Autodesk Inventor part; units mm, degrees
(part 3 of 4)
  line L942 (14.236161, -150.59225) -> (7.054859, -153.555032)
  spline S133 degree 3 poles (7.054859, -153.555032) (6.871236, -153.625657) (6.716206, -153.668031) (6.603207, -153.668031) (6.166024, -153.668031) (5.855277, -153.315254) (5.855277, -152.849821) (5.855277, -152.511168) (6.06715, -152.229015) (6.448178, -152.073641) knots 9 9 9 9 10 10 10 11 11 11 12 12 12 12
  line L943 (7.054859, -153.555032) -> (6.871236, -153.625657) construction
  line L944 (6.871236, -153.625657) -> (6.716206, -153.668031) construction
  line L945 (6.716206, -153.668031) -> (6.603207, -153.668031) construction
  line L946 (6.603207, -153.668031) -> (6.166024, -153.668031) construction
  line L947 (6.166024, -153.668031) -> (5.855277, -153.315254) construction
  line L948 (5.855277, -153.315254) -> (5.855277, -152.849821) construction
  line L949 (5.855277, -152.849821) -> (5.855277, -152.511168) construction
  line L950 (5.855277, -152.511168) -> (6.06715, -152.229015) construction
  line L951 (6.06715, -152.229015) -> (6.448178, -152.073641) construction
  line L952 (6.448178, -152.073641) -> (8.225847, -151.354305)
  line L953 (8.225847, -151.354305) -> (8.225847, -146.938037)
  line L954 (9.636614, -150.804124) -> (13.770384, -149.181484)
  line L955 (13.770384, -149.181484) -> (13.770384, -149.139109)
  line L956 (13.770384, -149.139109) -> (9.636614, -147.474439)
  line L957 (9.636614, -147.474439) -> (9.636614, -150.804124)
  spline S134 degree 3 poles (14.518314, -153.401381) (14.969621, -153.401381) (15.23765, -153.697659) (15.23765, -154.163436) knots 0 0 0 0 1 1 1 1
  line L958 (14.518314, -153.401381) -> (14.969621, -153.401381) construction
  line L959 (14.969621, -153.401381) -> (15.23765, -153.697659) construction
  line L960 (15.23765, -153.697659) -> (15.23765, -154.163436) construction
  line L961 (15.23765, -154.163436) -> (15.23765, -161.372988)
  spline S135 degree 3 poles (15.23765, -161.372988) (15.23765, -161.83842) (14.969621, -162.120573) (14.518314, -162.120573) (14.080787, -162.120573) (13.812758, -161.83842) (13.812758, -161.372988) knots 2 2 2 2 3 3 3 4 4 4 4
  line L962 (15.23765, -161.372988) -> (15.23765, -161.83842) construction
  line L963 (15.23765, -161.83842) -> (14.969621, -162.120573) construction
  line L964 (14.969621, -162.120573) -> (14.518314, -162.120573) construction
  line L965 (14.518314, -162.120573) -> (14.080787, -162.120573) construction
  line L966 (14.080787, -162.120573) -> (13.812758, -161.83842) construction
  line L967 (13.812758, -161.83842) -> (13.812758, -161.372988) construction
  line L968 (13.812758, -161.372988) -> (13.812758, -158.55111)
  line L969 (13.812758, -158.55111) -> (6.546708, -158.55111)
  spline S136 degree 3 poles (6.546708, -158.55111) (6.137775, -158.55111) (5.855277, -158.226582) (5.855277, -157.775274) (5.855277, -157.323622) (6.137775, -156.999094) (6.546708, -156.999094) knots 6 6 6 6 7 7 7 8 8 8 8
  line L970 (6.546708, -158.55111) -> (6.137775, -158.55111) construction
  line L971 (6.137775, -158.55111) -> (5.855277, -158.226582) construction
  line L972 (5.855277, -158.226582) -> (5.855277, -157.775274) construction
  line L973 (5.855277, -157.775274) -> (5.855277, -157.323622) construction
  line L974 (5.855277, -157.323622) -> (6.137775, -156.999094) construction
  line L975 (6.137775, -156.999094) -> (6.546708, -156.999094) construction
  line L976 (6.546708, -156.999094) -> (13.812758, -156.999094)
  line L977 (13.812758, -156.999094) -> (13.812758, -154.149311)
  spline S137 degree 3 poles (13.812758, -154.149311) (13.812758, -153.697659) (14.080787, -153.401381) (14.518314, -153.401381) knots 10 10 10 10 11 11 11 11
  line L978 (13.812758, -154.149311) -> (13.812758, -153.697659) construction
  line L979 (13.812758, -153.697659) -> (14.080787, -153.401381) construction
  line L980 (14.080787, -153.401381) -> (14.518314, -153.401381) construction
  spline S138 degree 3 poles (10.610198, -162.573603) (13.389701, -162.573603) (15.393024, -164.718175) (15.393024, -167.511803) (15.393024, -170.305431) (13.389701, -172.464128) (10.610198, -172.464128) (7.81657, -172.464128) (5.799122, -170.305431) (5.799122, -167.511803) (5.799122, -164.718175) (7.81657, -162.573603) (10.610198, -162.573603) knots 0 0 0 0 1 1 1 2 2 2 3 3 3 4 4 4 4
  line L981 (10.610198, -162.573603) -> (13.389701, -162.573603) construction
  line L982 (13.389701, -162.573603) -> (15.393024, -164.718175) construction
  line L983 (15.393024, -164.718175) -> (15.393024, -167.511803) construction
  line L984 (15.393024, -167.511803) -> (15.393024, -170.305431) construction
  line L985 (15.393024, -170.305431) -> (13.389701, -172.464128) construction
  line L986 (13.389701, -172.464128) -> (10.610198, -172.464128) construction
  line L987 (10.610198, -172.464128) -> (7.81657, -172.464128) construction
  line L988 (7.81657, -172.464128) -> (5.799122, -170.305431) construction
  line L989 (5.799122, -170.305431) -> (5.799122, -167.511803) construction
  line L990 (5.799122, -167.511803) -> (5.799122, -164.718175) construction
  line L991 (5.799122, -164.718175) -> (7.81657, -162.573603) construction
  line L992 (7.81657, -162.573603) -> (10.610198, -162.573603) construction
  spline S139 degree 3 poles (7.322888, -167.511803) (7.322888, -169.247098) (8.5645, -170.770863) (10.596073, -170.770863) (12.627646, -170.770863) (13.869258, -169.247098) (13.869258, -167.511803) (13.869258, -165.790633) (12.627646, -164.266868) (10.596073, -164.266868) (8.5645, -164.266868) (7.322888, -165.790633) (7.322888, -167.511803) knots 0 0 0 0 1 1 1 2 2 2 3 3 3 4 4 4 4
  line L993 (7.322888, -167.511803) -> (7.322888, -169.247098) construction
  line L994 (7.322888, -169.247098) -> (8.5645, -170.770863) construction
  line L995 (8.5645, -170.770863) -> (10.596073, -170.770863) construction
  line L996 (10.596073, -170.770863) -> (12.627646, -170.770863) construction
  line L997 (12.627646, -170.770863) -> (13.869258, -169.247098) construction
  line L998 (13.869258, -169.247098) -> (13.869258, -167.511803) construction
  line L999 (13.869258, -167.511803) -> (13.869258, -165.790633) construction
  line L1000 (13.869258, -165.790633) -> (12.627646, -164.266868) construction
  line L1001 (12.627646, -164.266868) -> (10.596073, -164.266868) construction
  line L1002 (10.596073, -164.266868) -> (8.5645, -164.266868) construction
  line L1003 (8.5645, -164.266868) -> (7.322888, -165.790633) construction
  line L1004 (7.322888, -165.790633) -> (7.322888, -167.511803) construction
  line L1005 (9.396835, -179.520028) -> (7.153389, -181.763474)
  spline S140 degree 3 poles (7.153389, -181.763474) (6.984235, -181.946753) (6.814736, -182.031503) (6.603207, -182.031503) (6.236304, -182.031503) (5.855277, -181.69285) (5.855277, -181.241198) (5.855277, -180.987294) (5.968276, -180.81814) (6.1519, -180.648641) knots 1 1 1 1 2 2 2 3 3 3 4 4 4 4
  line L1006 (7.153389, -181.763474) -> (6.984235, -181.946753) construction
  line L1007 (6.984235, -181.946753) -> (6.814736, -182.031503) construction
  line L1008 (6.814736, -182.031503) -> (6.603207, -182.031503) construction
  line L1009 (6.603207, -182.031503) -> (6.236304, -182.031503) construction
  line L1010 (6.236304, -182.031503) -> (5.855277, -181.69285) construction
  line L1011 (5.855277, -181.69285) -> (5.855277, -181.241198) construction
  line L1012 (5.855277, -181.241198) -> (5.855277, -180.987294) construction
  line L1013 (5.855277, -180.987294) -> (5.968276, -180.81814) construction
  line L1014 (5.968276, -180.81814) -> (6.1519, -180.648641) construction
  line L1015 (6.1519, -180.648641) -> (9.185306, -177.742359)
  line L1016 (9.185306, -177.742359) -> (9.185306, -176.162093)
  line L1017 (9.185306, -176.162093) -> (6.546708, -176.162093)
  spline S141 degree 3 poles (6.546708, -176.162093) (6.12365, -176.162093) (5.855277, -175.837565) (5.855277, -175.386258) (5.855277, -174.934606) (6.12365, -174.610078) (6.546708, -174.610078) knots 7 7 7 7 8 8 8 9 9 9 9
  line L1018 (6.546708, -176.162093) -> (6.12365, -176.162093) construction
  line L1019 (6.12365, -176.162093) -> (5.855277, -175.837565) construction
  line L1020 (5.855277, -175.837565) -> (5.855277, -175.386258) construction
  line L1021 (5.855277, -175.386258) -> (5.855277, -174.934606) construction
  line L1022 (5.855277, -174.934606) -> (6.12365, -174.610078) construction
  line L1023 (6.12365, -174.610078) -> (6.546708, -174.610078) construction
  line L1024 (6.546708, -174.610078) -> (14.574814, -174.610078)
  spline S142 degree 3 poles (14.574814, -174.610078) (14.983746, -174.610078) (15.23765, -174.864326) (15.23765, -175.315633) knots 10 10 10 10 11 11 11 11
  line L1025 (14.574814, -174.610078) -> (14.983746, -174.610078) construction
  line L1026 (14.983746, -174.610078) -> (15.23765, -174.864326) construction
  line L1027 (15.23765, -174.864326) -> (15.23765, -175.315633) construction
  line L1028 (15.23765, -175.315633) -> (15.23765, -178.221916)
  spline S143 degree 3 poles (15.23765, -178.221916) (15.23765, -180.81814) (13.826883, -181.904379) (12.303118, -181.904379) (11.160379, -181.904379) (9.777863, -181.199168) (9.396835, -179.520028) knots 12 12 12 12 13 13 13 14 14 14 14
  line L1029 (15.23765, -178.221916) -> (15.23765, -180.81814) construction
  line L1030 (15.23765, -180.81814) -> (13.826883, -181.904379) construction
  line L1031 (13.826883, -181.904379) -> (12.303118, -181.904379) construction
  line L1032 (12.303118, -181.904379) -> (11.160379, -181.904379) construction
  line L1033 (11.160379, -181.904379) -> (9.777863, -181.199168) construction
  line L1034 (9.777863, -181.199168) -> (9.396835, -179.520028) construction
  spline S144 degree 3 poles (10.581948, -178.109261) (10.581948, -179.661277) (11.315409, -180.211459) (12.204243, -180.211459) (13.079298, -180.211459) (13.812758, -179.661277) (13.812758, -178.109261) knots 0 0 0 0 1 1 1 2 2 2 2
  line L1035 (10.581948, -178.109261) -> (10.581948, -179.661277) construction
  line L1036 (10.581948, -179.661277) -> (11.315409, -180.211459) construction
  line L1037 (11.315409, -180.211459) -> (12.204243, -180.211459) construction
  line L1038 (12.204243, -180.211459) -> (13.079298, -180.211459) construction
  line L1039 (13.079298, -180.211459) -> (13.812758, -179.661277) construction
  line L1040 (13.812758, -179.661277) -> (13.812758, -178.109261) construction
  line L1041 (13.812758, -178.109261) -> (13.812758, -176.444247)
  spline S145 degree 3 poles (13.812758, -176.444247) (13.812758, -176.246843) (13.728009, -176.162093) (13.48823, -176.162093) knots 3 3 3 3 4 4 4 4
  line L1042 (13.812758, -176.444247) -> (13.812758, -176.246843) construction
  line L1043 (13.812758, -176.246843) -> (13.728009, -176.162093) construction
  line L1044 (13.728009, -176.162093) -> (13.48823, -176.162093) construction
  line L1045 (13.48823, -176.162093) -> (10.581948, -176.162093)
  line L1046 (10.581948, -176.162093) -> (10.581948, -178.109261)
  spline S146 degree 3 poles (5.855277, -187.535387) (5.855277, -187.09786) (6.12365, -186.759552) (6.546708, -186.759552) knots 0 0 0 0 1 1 1 1
  line L1047 (5.855277, -187.535387) -> (5.855277, -187.09786) construction
  line L1048 (5.855277, -187.09786) -> (6.12365, -186.759552) construction
  line L1049 (6.12365, -186.759552) -> (6.546708, -186.759552) construction
  line L1050 (6.546708, -186.759552) -> (9.664863, -186.759552)
  line L1051 (9.664863, -186.759552) -> (14.066662, -183.288618)
  spline S147 degree 3 poles (14.066662, -183.288618) (14.603063, -182.865216) (15.336524, -183.260368) (15.336524, -183.951799) (15.336524, -184.262202) (15.16737, -184.473731) (14.871092, -184.699385) knots 3 3 3 3 4 4 4 5 5 5 5
  line L1052 (14.066662, -183.288618) -> (14.603063, -182.865216) construction
  line L1053 (14.603063, -182.865216) -> (15.336524, -183.260368) construction
  line L1054 (15.336524, -183.260368) -> (15.336524, -183.951799) construction
  line L1055 (15.336524, -183.951799) -> (15.336524, -184.262202) construction
  line L1056 (15.336524, -184.262202) -> (15.16737, -184.473731) construction
  line L1057 (15.16737, -184.473731) -> (14.871092, -184.699385) construction
  line L1058 (14.871092, -184.699385) -> (11.231004, -187.549512)
  line L1059 (11.231004, -187.549512) -> (14.856967, -190.38517)
  spline S148 degree 3 poles (14.856967, -190.38517) (15.153245, -190.625293) (15.336524, -190.794447) (15.336524, -191.147225) (15.336524, -191.838656) (14.574814, -192.219339) (14.038412, -191.782156) knots 7 7 7 7 8 8 8 9 9 9 9
  line L1060 (14.856967, -190.38517) -> (15.153245, -190.625293) construction
  line L1061 (15.153245, -190.625293) -> (15.336524, -190.794447) construction
  line L1062 (15.336524, -190.794447) -> (15.336524, -191.147225) construction
  line L1063 (15.336524, -191.147225) -> (15.336524, -191.838656) construction
  line L1064 (15.336524, -191.838656) -> (14.574814, -192.219339) construction
  line L1065 (14.574814, -192.219339) -> (14.038412, -191.782156) construction
  line L1066 (14.038412, -191.782156) -> (9.678988, -188.311223)
  line L1067 (9.678988, -188.311223) -> (6.546708, -188.311223)
  spline S149 degree 3 poles (6.546708, -188.311223) (6.12365, -188.311223) (5.855277, -187.958789) (5.855277, -187.535387) knots 11 11 11 11 12 12 12 12
  line L1068 (6.546708, -188.311223) -> (6.12365, -188.311223) construction
  line L1069 (6.12365, -188.311223) -> (5.855277, -187.958789) construction
  line L1070 (5.855277, -187.958789) -> (5.855277, -187.535387) construction
  line L1071 (6.400291, -6.445968) -> (12.750291, -6.445968) construction
  line L1072 (46.338938, -27.465197) -> (52.688938, -27.465197) construction
  line L1073 (47.834799, -200.192668) -> (54.184799, -200.192668) construction
  line L1074 (5.855277, -187.958789) -> (12.205277, -187.958789) construction
  line L1075 (1.910163, -1.95584) -> (1.910163, -192.45584)
  line L1076 (1.910163, -192.45584) -> (52.688938, -216.134372)
  line L1077 (52.688938, -216.134372) -> (52.450732, -216.645207)
  line L1078 (1.910163, -1.95584) -> (52.688938, -25.634372)
  line L1079 (1.910163, -1.95584) -> (57.938343, -1.95584) construction
  line L1080 (52.688938, -25.634372) -> (52.688938, -216.134372)
  point P0 (0, 0)
  point P1 (3.752764, -91.883884)
  dimension "d0" = 21.844
  dimension "d8" = 190.5
  dimension "d9" = 115
  dimension "d10" = 25
  constraints: 464 end point, 5 horizontal, 2 coincident, 2 vertical, 1 equal length, 1 perpendicular, 434 other
  measures "d0" distance of L5.start L1075.start
  measures "d8" distance of L1075.start L1075.end
  measures "d9" angle of L1076 L1075
  measures "d10" angle of L1078 L1079
sketch "Sketch1 outline for Extrusion1" plane through (0, 0, 0) normal (0, 1, 0) x (-1, 0, 0)
  line L0 (1.910163, -1.95584) -> (1.910163, -192.45584)
  line L1 (52.688938, -25.634372) -> (1.910163, -1.95584)
  line L2 (1.910163, -192.45584) -> (52.688938, -216.134372)
  line L3 (52.688938, -216.134372) -> (52.688938, -25.634372)
  spline S0 degree 3 poles (14.856967, -190.38517) (15.153245, -190.625293) (15.336524, -190.794447) (15.336524, -191.147225) (15.336524, -191.838656) (14.574814, -192.219339) (14.038412, -191.782156) knots 0 0 0 0 0.5 0.5 0.5 1 1 1 1
  line L4 (11.231004, -187.549512) -> (14.856967, -190.38517)
  line L5 (14.871092, -184.699385) -> (11.231004, -187.549512)
  spline S1 degree 3 poles (14.066662, -183.288618) (14.603063, -182.865216) (15.336524, -183.260368) (15.336524, -183.951799) (15.336524, -184.262202) (15.16737, -184.473731) (14.871092, -184.699385) knots 0 0 0 0 0.5 0.5 0.5 1 1 1 1
  line L6 (9.664863, -186.759552) -> (14.066662, -183.288618)
  line L7 (6.546708, -186.759552) -> (9.664863, -186.759552)
  spline S2 degree 3 poles (5.855277, -187.535387) (5.855277, -187.09786) (6.12365, -186.759552) (6.546708, -186.759552) knots 0 0 0 0 1 1 1 1
  spline S3 degree 3 poles (6.546708, -188.311223) (6.12365, -188.311223) (5.855277, -187.958789) (5.855277, -187.535387) knots 0 0 0 0 1 1 1 1
  line L8 (9.678988, -188.311223) -> (6.546708, -188.311223)
  line L9 (14.038412, -191.782156) -> (9.678988, -188.311223)
  spline S4 degree 3 poles (6.546708, -176.162093) (6.12365, -176.162093) (5.855277, -175.837565) (5.855277, -175.386258) (5.855277, -174.934606) (6.12365, -174.610078) (6.546708, -174.610078) knots 0 0 0 0 0.5 0.5 0.5 1 1 1 1
  line L10 (9.185306, -176.162093) -> (6.546708, -176.162093)
  line L11 (9.185306, -177.742359) -> (9.185306, -176.162093)
  line L12 (6.1519, -180.648641) -> (9.185306, -177.742359)
  spline S5 degree 3 poles (7.153389, -181.763474) (6.984235, -181.946753) (6.814736, -182.031503) (6.603207, -182.031503) (6.236304, -182.031503) (5.855277, -181.69285) (5.855277, -181.241198) (5.855277, -180.987294) (5.968276, -180.81814) (6.1519, -180.648641) knots 0 0 0 0 0.33333333 0.33333333 0.33333333 0.66666667 0.66666667 0.66666667 1 1 1 1
  line L13 (9.396835, -179.520028) -> (7.153389, -181.763474)
  spline S6 degree 3 poles (15.23765, -178.221916) (15.23765, -180.81814) (13.826883, -181.904379) (12.303118, -181.904379) (11.160379, -181.904379) (9.777863, -181.199168) (9.396835, -179.520028) knots 0 0 0 0 0.5 0.5 0.5 1 1 1 1
  line L14 (15.23765, -175.315633) -> (15.23765, -178.221916)
  spline S7 degree 3 poles (14.574814, -174.610078) (14.983746, -174.610078) (15.23765, -174.864326) (15.23765, -175.315633) knots 0 0 0 0 1 1 1 1
  line L15 (6.546708, -174.610078) -> (14.574814, -174.610078)
  spline S8 degree 3 poles (10.610198, -162.573603) (13.389701, -162.573603) (15.393024, -164.718175) (15.393024, -167.511803) (15.393024, -170.305431) (13.389701, -172.464128) (10.610198, -172.464128) (7.81657, -172.464128) (5.799122, -170.305431) (5.799122, -167.511803) (5.799122, -164.718175) (7.81657, -162.573603) (10.610198, -162.573603) knots 0 0 0 0 0.25 0.25 0.25 0.5 0.5 0.5 0.75 0.75 0.75 1 1 1 1
  spline S9 degree 3 poles (13.812758, -154.149311) (13.812758, -153.697659) (14.080787, -153.401381) (14.518314, -153.401381) knots 0 0 0 0 1 1 1 1
  line L16 (13.812758, -156.999094) -> (13.812758, -154.149311)
  line L17 (6.546708, -156.999094) -> (13.812758, -156.999094)
  spline S10 degree 3 poles (6.546708, -158.55111) (6.137775, -158.55111) (5.855277, -158.226582) (5.855277, -157.775274) (5.855277, -157.323622) (6.137775, -156.999094) (6.546708, -156.999094) knots 0 0 0 0 0.5 0.5 0.5 1 1 1 1
  line L18 (13.812758, -158.55111) -> (6.546708, -158.55111)
  line L19 (13.812758, -161.372988) -> (13.812758, -158.55111)
  spline S11 degree 3 poles (15.23765, -161.372988) (15.23765, -161.83842) (14.969621, -162.120573) (14.518314, -162.120573) (14.080787, -162.120573) (13.812758, -161.83842) (13.812758, -161.372988) knots 0 0 0 0 0.5 0.5 0.5 1 1 1 1
  line L20 (15.23765, -154.163436) -> (15.23765, -161.372988)
  spline S12 degree 3 poles (14.518314, -153.401381) (14.969621, -153.401381) (15.23765, -153.697659) (15.23765, -154.163436) knots 0 0 0 0 1 1 1 1
  line L21 (8.225847, -146.938037) -> (6.434053, -146.204577)
  line L22 (8.225847, -151.354305) -> (8.225847, -146.938037)
  line L23 (6.448178, -152.073641) -> (8.225847, -151.354305)
  spline S13 degree 3 poles (7.054859, -153.555032) (6.871236, -153.625657) (6.716206, -153.668031) (6.603207, -153.668031) (6.166024, -153.668031) (5.855277, -153.315254) (5.855277, -152.849821) (5.855277, -152.511168) (6.06715, -152.229015) (6.448178, -152.073641) knots 0 0 0 0 0.33333333 0.33333333 0.33333333 0.66666667 0.66666667 0.66666667 1 1 1 1
  line L24 (14.236161, -150.59225) -> (7.054859, -153.555032)
  spline S14 degree 3 poles (15.322399, -149.209733) (15.322399, -149.858789) (15.026121, -150.267722) (14.236161, -150.59225) knots 0 0 0 0 1 1 1 1
  line L25 (15.322399, -149.110859) -> (15.322399, -149.209733)
  spline S15 degree 3 poles (14.236161, -147.742467) (15.026121, -148.05287) (15.322399, -148.475928) (15.322399, -149.110859) knots 0 0 0 0 1 1 1 1
  line L26 (7.111014, -144.779685) -> (14.236161, -147.742467)
  spline S16 degree 3 poles (6.560832, -144.652561) (6.744456, -144.638436) (6.91361, -144.694936) (7.111014, -144.779685) knots 0 0 0 0 1 1 1 1
  spline S17 degree 3 poles (6.434053, -146.204577) (6.053025, -146.049203) (5.855277, -145.809424) (5.855277, -145.442521) (5.855277, -144.991214) (6.1519, -144.680811) (6.560832, -144.652561) knots 0 0 0 0 0.5 0.5 0.5 1 1 1 1
  line L27 (9.396835, -140.799222) -> (7.153389, -143.042668)
  spline S18 degree 3 poles (15.23765, -139.501454) (15.23765, -142.097334) (13.826883, -143.183572) (12.303118, -143.183572) (11.160379, -143.183572) (9.777863, -142.478361) (9.396835, -140.799222) knots 0 0 0 0 0.5 0.5 0.5 1 1 1 1
  line L28 (15.23765, -136.594827) -> (15.23765, -139.501454)
  spline S19 degree 3 poles (14.574814, -135.889616) (14.983746, -135.889616) (15.23765, -136.14352) (15.23765, -136.594827) knots 0 0 0 0 1 1 1 1
  line L29 (6.546708, -135.889616) -> (14.574814, -135.889616)
  spline S20 degree 3 poles (6.546708, -137.441632) (6.12365, -137.441632) (5.855277, -137.117104) (5.855277, -136.665452) (5.855277, -136.214144) (6.12365, -135.889616) (6.546708, -135.889616) knots 0 0 0 0 0.5 0.5 0.5 1 1 1 1
  line L30 (9.185306, -137.441632) -> (6.546708, -137.441632)
  line L31 (9.185306, -139.021553) -> (9.185306, -137.441632)
  line L32 (6.1519, -141.92818) -> (9.185306, -139.021553)
  spline S21 degree 3 poles (7.153389, -143.042668) (6.984235, -143.225947) (6.814736, -143.310696) (6.603207, -143.310696) (6.236304, -143.310696) (5.855277, -142.972044) (5.855277, -142.520736) (5.855277, -142.266832) (5.968276, -142.097334) (6.1519, -141.92818) knots 0 0 0 0 0.33333333 0.33333333 0.33333333 0.66666667 0.66666667 0.66666667 1 1 1 1
  spline S22 degree 3 poles (10.610198, -123.853142) (13.389701, -123.853142) (15.393024, -125.997714) (15.393024, -128.790997) (15.393024, -131.584625) (13.389701, -133.743322) (10.610198, -133.743322) (7.81657, -133.743322) (5.799122, -131.584625) (5.799122, -128.790997) (5.799122, -125.997714) (7.81657, -123.853142) (10.610198, -123.853142) knots 0 0 0 0 0.25 0.25 0.25 0.5 0.5 0.5 0.75 0.75 0.75 1 1 1 1
  spline S23 degree 3 poles (5.954151, -115.696706) (5.954151, -115.245226) (6.208055, -114.991322) (6.631457, -114.991322) knots 0 0 0 0 1 1 1 1
  line L33 (5.954151, -119.068593) -> (5.954151, -115.696706)
  spline S24 degree 3 poles (10.553698, -120.747733) (10.215045, -121.819846) (9.35446, -122.355903) (8.493876, -122.355903) (7.040734, -122.355903) (5.954151, -121.19904) (5.954151, -119.068593) knots 0 0 0 0 0.5 0.5 0.5 1 1 1 1
  spline S25 degree 3 poles (15.23765, -118.70169) (15.23765, -120.959261) (14.123162, -122.102) (12.599396, -122.102) (11.668186, -122.102) (10.864101, -121.509443) (10.553698, -120.747733) knots 0 0 0 0 0.5 0.5 0.5 1 1 1 1
  line L34 (15.23765, -115.696706) -> (15.23765, -118.70169)
  spline S26 degree 3 poles (14.574814, -114.991322) (14.983746, -114.991322) (15.23765, -115.245226) (15.23765, -115.696706) knots 0 0 0 0 1 1 1 1
  line L35 (6.631457, -114.991322) -> (14.574814, -114.991322)
  line L36 (29.80093, -191.867595) -> (23.480041, -191.867595)
  line L37 (23.494166, -196.368267) -> (29.80093, -191.867595)
  spline S27 degree 3 poles (22.788955, -197.51135) (22.788955, -197.031448) (23.000484, -196.721045) (23.494166, -196.368267) knots 0 0 0 0 1 1 1 1
  line L38 (22.788955, -197.567505) -> (22.788955, -197.51135)
  spline S28 degree 3 poles (23.62129, -198.498714) (23.127263, -198.498714) (22.788955, -198.061532) (22.788955, -197.567505) knots 0 0 0 0 1 1 1 1
  line L39 (31.578599, -198.498714) -> (23.62129, -198.498714)
  spline S29 degree 3 poles (31.578599, -196.946699) (31.987876, -196.946699) (32.27003, -197.271227) (32.27003, -197.722879) (32.27003, -198.174187) (31.987876, -198.498714) (31.578599, -198.498714) knots 0 0 0 0 0.5 0.5 0.5 1 1 1 1
  line L40 (25.356757, -196.946699) -> (31.578599, -196.946699)
  line L41 (31.479897, -192.446026) -> (25.356757, -196.946699)
  spline S30 degree 3 poles (32.255905, -191.260913) (32.255905, -191.740815) (32.086578, -191.994719) (31.479897, -192.446026) knots 0 0 0 0 1 1 1 1
  line L42 (32.255905, -191.176509) -> (32.255905, -191.260913)
  spline S31 degree 3 poles (31.324696, -190.315579) (31.889002, -190.315579) (32.255905, -190.696607) (32.255905, -191.176509) knots 0 0 0 0 1 1 1 1
  line L43 (23.480041, -190.315579) -> (31.324696, -190.315579)
  spline S32 degree 3 poles (23.480041, -191.867595) (23.071108, -191.867595) (22.788955, -191.543067) (22.788955, -191.091759) (22.788955, -190.640107) (23.071108, -190.315579) (23.480041, -190.315579) knots 0 0 0 0 0.5 0.5 0.5 1 1 1 1
  spline S33 degree 3 poles (27.543531, -178.279105) (30.323034, -178.279105) (32.326357, -180.423677) (32.326357, -183.217304) (32.326357, -186.010932) (30.323034, -188.169629) (27.543531, -188.169629) (24.750075, -188.169629) (22.732455, -186.010932) (22.732455, -183.217304) (22.732455, -180.423677) (24.750075, -178.279105) (27.543531, -178.279105) knots 0 0 0 0 0.25 0.25 0.25 0.5 0.5 0.5 0.75 0.75 0.75 1 1 1 1
  spline S34 degree 3 poles (31.578599, -174.595953) (31.987876, -174.595953) (32.27003, -174.920481) (32.27003, -175.372133) knots 0 0 0 0 1 1 1 1
  line L44 (23.480041, -174.595953) -> (31.578599, -174.595953)
  spline S35 degree 3 poles (23.480041, -176.147969) (23.071108, -176.147969) (22.788955, -175.823441) (22.788955, -175.372133) (22.788955, -174.920481) (23.071108, -174.595953) (23.480041, -174.595953) knots 0 0 0 0 0.5 0.5 0.5 1 1 1 1
  line L45 (31.578599, -176.147969) -> (23.480041, -176.147969)
  spline S36 degree 3 poles (32.27003, -175.372133) (32.27003, -175.823441) (31.987876, -176.147969) (31.578599, -176.147969) knots 0 0 0 0 1 1 1 1
  line L46 (30.746264, -169.444846) -> (23.480041, -169.444846)
  line L47 (30.746264, -172.266724) -> (30.746264, -169.444846)
  spline S37 degree 3 poles (32.171155, -172.266724) (32.171155, -172.732156) (31.903127, -173.01431) (31.451647, -173.01431) (31.014292, -173.01431) (30.746264, -172.732156) (30.746264, -172.266724) knots 0 0 0 0 0.5 0.5 0.5 1 1 1 1
  line L48 (32.171155, -165.057173) -> (32.171155, -172.266724)
  spline S38 degree 3 poles (31.451647, -164.295117) (31.903127, -164.295117) (32.171155, -164.591396) (32.171155, -165.057173) knots 0 0 0 0 1 1 1 1
  spline S39 degree 3 poles (30.746264, -165.043048) (30.746264, -164.591396) (31.014292, -164.295117) (31.451647, -164.295117) knots 0 0 0 0 1 1 1 1
  line L49 (30.746264, -167.892831) -> (30.746264, -165.043048)
  line L50 (23.480041, -167.892831) -> (30.746264, -167.892831)
  spline S40 degree 3 poles (23.480041, -169.444846) (23.071108, -169.444846) (22.788955, -169.120318) (22.788955, -168.669011) (22.788955, -168.217359) (23.071108, -167.892831) (23.480041, -167.892831) knots 0 0 0 0 0.5 0.5 0.5 1 1 1 1
  line L51 (25.15918, -162.248042) -> (25.15918, -157.831774)
  line L52 (23.381511, -162.967378) -> (25.15918, -162.248042)
  spline S41 degree 3 poles (23.988192, -164.448769) (23.804569, -164.519393) (23.64954, -164.561768) (23.53654, -164.561768) (23.099358, -164.561768) (22.788955, -164.20899) (22.788955, -163.743558) (22.788955, -163.404905) (23.000484, -163.122752) (23.381511, -162.967378) knots 0 0 0 0 0.33333333 0.33333333 0.33333333 0.66666667 0.66666667 0.66666667 1 1 1 1
  line L53 (31.169494, -161.485987) -> (23.988192, -164.448769)
  spline S42 degree 3 poles (32.255905, -160.10347) (32.255905, -160.752526) (31.959627, -161.161459) (31.169494, -161.485987) knots 0 0 0 0 1 1 1 1
  line L54 (32.255905, -160.004596) -> (32.255905, -160.10347)
  spline S43 degree 3 poles (31.169494, -158.636204) (31.959627, -158.946607) (32.255905, -159.369664) (32.255905, -160.004596) knots 0 0 0 0 1 1 1 1
  line L55 (24.044348, -155.673422) -> (31.169494, -158.636204)
  spline S44 degree 3 poles (23.494166, -155.546298) (23.677789, -155.532173) (23.846944, -155.588672) (24.044348, -155.673422) knots 0 0 0 0 1 1 1 1
  spline S45 degree 3 poles (23.367386, -157.098313) (22.986359, -156.942939) (22.788955, -156.703161) (22.788955, -156.336258) (22.788955, -155.88495) (23.085233, -155.574547) (23.494166, -155.546298) knots 0 0 0 0 0.5 0.5 0.5 1 1 1 1
  line L56 (25.15918, -157.831774) -> (23.367386, -157.098313)
  spline S46 degree 3 poles (48.511932, -199.684861) (48.356731, -199.938764) (48.159327, -200.192668) (47.834799, -200.192668) (47.453771, -200.192668) (47.072916, -199.952889) (47.072916, -199.515707) (47.072916, -199.289708) (47.129243, -199.148804) (47.242242, -198.937275) (47.524396, -198.344374) (47.792424, -197.540289) (47.792424, -196.679704) (47.792424, -195.325437) (47.171618, -194.577507) (46.466235, -194.577507) (45.520901, -194.577507) (45.281122, -195.494591) (44.956594, -197.159261) (44.617941, -198.866651) (44.251211, -200.418666) (42.360542, -200.418666) (40.879151, -200.418666) (39.651664, -199.02168) (39.651664, -196.707954) (39.651664, -195.212438) (40.117268, -193.815796) (40.596998, -193.081991) (40.794574, -192.799838) (41.048478, -192.729213) (41.231929, -192.729213) (41.641034, -192.729213) (42.036014, -193.039616) (42.036014, -193.448894) (42.036014, -193.646298) (41.951437, -193.843701) (41.852563, -194.04145) (41.457583, -194.83141) (41.161304, -195.790869) (41.161304, -196.792703) (41.161304, -198.076346) (41.626909, -198.767776) (42.332292, -198.767776) (43.1083, -198.767776) (43.305876, -198.020191) (43.644529, -196.312801) (43.98301, -194.591632) (44.364037, -192.926617) (46.437985, -192.926617) (47.877001, -192.926617) (49.25969, -194.238854) (49.25969, -196.750329) (49.25969, -198.006066) (48.808211, -199.191179) (48.511932, -199.684861) knots 0 0 0 0 0.05555556 0.05555556 0.05555556 0.11111111 0.11111111 0.11111111 0.16666667 0.16666667 0.16666667 0.22222222 0.22222222 0.22222222 0.27777778 0.27777778 0.27777778 0.33333333 0.33333333 0.33333333 0.38888889 0.38888889 0.38888889 0.44444444 0.44444444 0.44444444 0.5 0.5 0.5 0.55555556 0.55555556 0.55555556 0.61111111 0.61111111 0.61111111 0.66666667 0.66666667 0.66666667 0.72222222 0.72222222 0.72222222 0.77777778 0.77777778 0.77777778 0.83333333 0.83333333 0.83333333 0.88888889 0.88888889 0.88888889 0.94444444 0.94444444 0.94444444 1 1 1 1
  line L57 (48.511932, -184.121298) -> (43.785606, -184.121298)
  spline S47 degree 3 poles (48.511932, -182.569282) (48.92121, -182.569282) (49.203363, -182.89381) (49.203363, -183.345117) (49.203363, -183.79677) (48.92121, -184.121298) (48.511932, -184.121298) knots 0 0 0 0 0.5 0.5 0.5 1 1 1 1
  line L58 (43.700857, -182.569282) -> (48.511932, -182.569282)
  spline S48 degree 3 poles (43.700857, -190.582919) (41.358881, -190.582919) (39.637539, -189.087403) (39.637539, -186.575928) (39.637539, -184.050673) (41.358881, -182.569282) (43.700857, -182.569282) knots 0 0 0 0 0.5 0.5 0.5 1 1 1 1
  line L59 (48.511932, -190.582919) -> (43.700857, -190.582919)
  spline S49 degree 3 poles (48.511932, -189.030903) (48.92121, -189.030903) (49.203363, -189.355431) (49.203363, -189.807083) (49.203363, -190.258391) (48.92121, -190.582919) (48.511932, -190.582919) knots 0 0 0 0 0.5 0.5 0.5 1 1 1 1
  line L60 (43.785606, -189.030903) -> (48.511932, -189.030903)
  spline S50 degree 3 poles (41.14718, -186.575928) (41.14718, -188.085569) (42.177091, -189.030903) (43.785606, -189.030903) knots 0 0 0 0 1 1 1 1
  spline S51 degree 3 poles (43.785606, -184.121298) (42.191216, -184.121298) (41.14718, -185.052162) (41.14718, -186.575928) knots 0 0 0 0 1 1 1 1
  spline S52 degree 3 poles (44.476864, -170.617212) (47.256367, -170.617212) (49.25969, -172.761784) (49.25969, -175.555412) (49.25969, -178.34904) (47.256367, -180.507737) (44.476864, -180.507737) (41.683409, -180.507737) (39.665788, -178.34904) (39.665788, -175.555412) (39.665788, -172.761784) (41.683409, -170.617212) (44.476864, -170.617212) knots 0 0 0 0 0.25 0.25 0.25 0.5 0.5 0.5 0.75 0.75 0.75 1 1 1 1
  line L61 (46.706013, -166.890652) -> (43.729106, -164.858735)
  line L62 (46.706013, -166.918902) -> (46.706013, -166.890652)
  line L63 (40.413546, -166.918902) -> (46.706013, -166.918902)
  spline S53 degree 3 poles (40.413546, -168.470918) (39.990316, -168.470918) (39.722288, -168.14639) (39.722288, -167.694738) (39.722288, -167.24343) (39.990316, -166.918902) (40.413546, -166.918902) knots 0 0 0 0 0.5 0.5 0.5 1 1 1 1
  line L64 (48.286279, -168.470918) -> (40.413546, -168.470918)
  spline S54 degree 3 poles (49.189238, -167.567958) (49.189238, -168.075765) (48.83646, -168.470918) (48.286279, -168.470918) knots 0 0 0 0 1 1 1 1
  line L65 (49.189238, -167.454959) -> (49.189238, -167.567958)
  spline S55 degree 3 poles (48.455605, -166.36872) (48.86471, -166.650874) (49.189238, -166.918902) (49.189238, -167.454959) knots 0 0 0 0 1 1 1 1
  line L66 (44.998969, -164.0264) -> (48.455605, -166.36872)
  line L67 (44.998969, -164.012275) -> (44.998969, -164.0264)
  line L68 (48.44148, -161.656174) -> (44.998969, -164.012275)
  spline S56 degree 3 poles (49.189238, -160.499311) (49.189238, -161.035368) (48.86471, -161.374021) (48.44148, -161.656174) knots 0 0 0 0 1 1 1 1
  line L69 (49.189238, -160.386312) -> (49.189238, -160.499311)
  spline S57 degree 3 poles (48.286279, -159.469228) (48.83646, -159.469228) (49.189238, -159.86438) (49.189238, -160.386312) knots 0 0 0 0 1 1 1 1
  line L70 (40.413546, -159.469228) -> (48.286279, -159.469228)
  spline S58 degree 3 poles (40.413546, -161.021243) (39.990316, -161.021243) (39.722288, -160.696715) (39.722288, -160.245408) (39.722288, -159.793756) (39.990316, -159.469228) (40.413546, -159.469228) knots 0 0 0 0 0.5 0.5 0.5 1 1 1 1
  line L71 (46.706013, -161.021243) -> (40.413546, -161.021243)
  line L72 (46.706013, -161.063618) -> (46.706013, -161.021243)
  line L73 (43.729106, -163.095191) -> (46.706013, -161.063618)
  spline S59 degree 3 poles (43.729106, -164.858735) (43.305876, -164.576582) (43.13655, -164.350928) (43.13655, -163.9699) (43.13655, -163.602998) (43.305876, -163.391469) (43.729106, -163.095191) knots 0 0 0 0 0.5 0.5 0.5 1 1 1 1
  line L74 (31.578599, -149.53495) -> (24.651201, -149.53495)
  spline S60 degree 3 poles (32.255905, -148.75877) (32.255905, -149.210422) (31.987876, -149.53495) (31.578599, -149.53495) knots 0 0 0 0 1 1 1 1
  spline S61 degree 3 poles (31.578599, -147.982935) (31.987876, -147.982935) (32.255905, -148.307463) (32.255905, -148.75877) knots 0 0 0 0 1 1 1 1
  line L75 (23.607165, -147.982935) -> (31.578599, -147.982935)
  spline S62 degree 3 poles (22.887484, -148.744645) (22.887484, -148.279213) (23.141388, -147.982935) (23.607165, -147.982935) knots 0 0 0 0 1 1 1 1
  line L76 (22.887484, -153.936749) -> (22.887484, -148.744645)
  spline S63 degree 3 poles (24.326501, -153.936749) (24.326501, -154.402181) (24.058472, -154.684335) (23.607165, -154.684335) (23.155513, -154.684335) (22.887484, -154.402181) (22.887484, -153.936749) knots 0 0 0 0 0.5 0.5 0.5 1 1 1 1
  line L77 (24.326501, -149.817104) -> (24.326501, -153.936749)
  spline S64 degree 3 poles (24.651201, -149.53495) (24.397125, -149.53495) (24.326501, -149.619355) (24.326501, -149.817104) knots 0 0 0 0 1 1 1 1
  spline S65 degree 3 poles (24.213846, -141.321843) (24.213846, -142.831484) (25.243757, -143.776818) (26.852273, -143.776818) knots 0 0 0 0 1 1 1 1
  spline S66 degree 3 poles (26.852273, -138.866868) (25.257882, -138.866868) (24.213846, -139.798077) (24.213846, -141.321843) knots 0 0 0 0 1 1 1 1
  line L78 (31.578599, -138.866868) -> (26.852273, -138.866868)
  spline S67 degree 3 poles (31.578599, -137.314852) (31.987876, -137.314852) (32.27003, -137.63938) (32.27003, -138.090688) (32.27003, -138.54234) (31.987876, -138.866868) (31.578599, -138.866868) knots 0 0 0 0 0.5 0.5 0.5 1 1 1 1
  line L79 (26.767523, -137.314852) -> (31.578599, -137.314852)
  spline S68 degree 3 poles (26.767523, -145.328489) (24.425375, -145.328489) (22.704205, -143.832973) (22.704205, -141.321843) (22.704205, -138.796243) (24.425375, -137.314852) (26.767523, -137.314852) knots 0 0 0 0 0.5 0.5 0.5 1 1 1 1
  line L80 (31.578599, -145.328489) -> (26.767523, -145.328489)
  spline S69 degree 3 poles (31.578599, -143.776818) (31.987876, -143.776818) (32.27003, -144.101001) (32.27003, -144.552653) (32.27003, -145.003961) (31.987876, -145.328489) (31.578599, -145.328489) knots 0 0 0 0 0.5 0.5 0.5 1 1 1 1
  line L81 (26.852273, -143.776818) -> (31.578599, -143.776818)
  line L82 (29.77268, -133.108735) -> (29.77268, -133.080485)
  line L83 (23.480041, -133.108735) -> (29.77268, -133.108735)
  spline S70 degree 3 poles (23.480041, -134.660751) (23.056983, -134.660751) (22.788955, -134.336223) (22.788955, -133.884571) (22.788955, -133.433263) (23.056983, -133.108735) (23.480041, -133.108735) knots 0 0 0 0 0.5 0.5 0.5 1 1 1 1
  line L84 (31.352945, -134.660751) -> (23.480041, -134.660751)
  spline S71 degree 3 poles (32.255905, -133.757791) (32.255905, -134.265598) (31.903127, -134.660751) (31.352945, -134.660751) knots 0 0 0 0 1 1 1 1
  line L85 (32.255905, -133.644792) -> (32.255905, -133.757791)
  spline S72 degree 3 poles (31.522272, -132.558553) (31.931377, -132.840707) (32.255905, -133.108735) (32.255905, -133.644792) knots 0 0 0 0 1 1 1 1
  line L86 (28.065635, -130.216577) -> (31.522272, -132.558553)
  line L87 (28.065635, -130.202453) -> (28.065635, -130.216577)
  line L88 (31.508147, -127.846007) -> (28.065635, -130.202453)
  spline S73 degree 3 poles (32.255905, -126.689144) (32.255905, -127.225546) (31.931377, -127.563854) (31.508147, -127.846007) knots 0 0 0 0 1 1 1 1
  line L89 (32.255905, -126.57649) -> (32.255905, -126.689144)
  spline S74 degree 3 poles (31.352945, -125.659405) (31.903127, -125.659405) (32.255905, -126.054213) (32.255905, -126.57649) knots 0 0 0 0 1 1 1 1
  line L90 (23.480041, -125.659405) -> (31.352945, -125.659405)
  spline S75 degree 3 poles (23.480041, -127.211421) (23.056983, -127.211421) (22.788955, -126.886893) (22.788955, -126.435241) (22.788955, -125.983933) (23.056983, -125.659405) (23.480041, -125.659405) knots 0 0 0 0 0.5 0.5 0.5 1 1 1 1
  line L91 (29.77268, -127.211421) -> (23.480041, -127.211421)
  line L92 (29.77268, -127.253451) -> (29.77268, -127.211421)
  line L93 (26.795773, -129.285368) -> (29.77268, -127.253451)
  spline S76 degree 3 poles (26.795773, -131.048913) (26.372543, -130.766759) (26.203217, -130.540761) (26.203217, -130.160078) (26.203217, -129.793175) (26.372543, -129.581646) (26.795773, -129.285368) knots 0 0 0 0 0.5 0.5 0.5 1 1 1 1
  line L94 (29.77268, -133.080485) -> (26.795773, -131.048913)
  line L95 (26.118639, -119.196062) -> (26.118639, -117.615968)
  line L96 (23.085233, -122.102344) -> (26.118639, -119.196062)
  spline S77 degree 3 poles (24.086722, -123.216832) (23.917568, -123.400456) (23.748069, -123.485205) (23.53654, -123.485205) (23.169638, -123.485205) (22.788955, -123.146553) (22.788955, -122.6949) (22.788955, -122.440997) (22.901609, -122.271843) (23.085233, -122.102344) knots 0 0 0 0 0.33333333 0.33333333 0.33333333 0.66666667 0.66666667 0.66666667 1 1 1 1
  line L97 (26.330168, -120.973731) -> (24.086722, -123.216832)
  spline S78 degree 3 poles (32.171155, -119.675619) (32.171155, -122.271843) (30.760389, -123.358081) (29.236623, -123.358081) (28.093713, -123.358081) (26.711196, -122.652526) (26.330168, -120.973731) knots 0 0 0 0 0.5 0.5 0.5 1 1 1 1
  line L98 (32.171155, -116.769336) -> (32.171155, -119.675619)
  spline S79 degree 3 poles (31.508147, -116.063953) (31.917252, -116.063953) (32.171155, -116.317856) (32.171155, -116.769336) knots 0 0 0 0 1 1 1 1
  line L99 (23.480041, -116.063953) -> (31.508147, -116.063953)
  spline S80 degree 3 poles (23.480041, -117.615968) (23.056983, -117.615968) (22.788955, -117.29144) (22.788955, -116.839961) (22.788955, -116.388481) (23.056983, -116.063953) (23.480041, -116.063953) knots 0 0 0 0 0.5 0.5 0.5 1 1 1 1
  line L100 (26.118639, -117.615968) -> (23.480041, -117.615968)
  spline S81 degree 3 poles (44.476864, -147.432753) (47.256367, -147.432753) (49.25969, -149.577325) (49.25969, -152.370953) (49.25969, -155.164236) (47.256367, -157.322933) (44.476864, -157.322933) (41.683409, -157.322933) (39.665788, -155.164236) (39.665788, -152.370953) (39.665788, -149.577325) (41.683409, -147.432753) (44.476864, -147.432753) knots 0 0 0 0 0.25 0.25 0.25 0.5 0.5 0.5 0.75 0.75 0.75 1 1 1 1
  spline S82 degree 3 poles (40.413546, -138.655683) (40.004441, -138.655683) (39.722288, -138.331155) (39.722288, -137.879503) (39.722288, -137.428196) (40.004441, -137.103668) (40.413546, -137.103668) knots 0 0 0 0 0.5 0.5 0.5 1 1 1 1
  line L101 (46.734263, -138.655683) -> (40.413546, -138.655683)
  line L102 (40.427671, -143.156356) -> (46.734263, -138.655683)
  spline S83 degree 3 poles (39.722288, -144.299094) (39.722288, -143.819192) (39.933817, -143.508789) (40.427671, -143.156356) knots 0 0 0 0 1 1 1 1
  line L103 (39.722288, -144.355594) -> (39.722288, -144.299094)
  spline S84 degree 3 poles (40.554623, -145.286803) (40.060769, -145.286803) (39.722288, -144.849276) (39.722288, -144.355594) knots 0 0 0 0 1 1 1 1
  line L104 (48.511932, -145.286803) -> (40.554623, -145.286803)
  spline S85 degree 3 poles (48.511932, -143.734788) (48.92121, -143.734788) (49.203363, -144.059316) (49.203363, -144.510623) (49.203363, -144.962275) (48.92121, -145.286803) (48.511932, -145.286803) knots 0 0 0 0 0.5 0.5 0.5 1 1 1 1
  line L105 (42.29009, -143.734788) -> (48.511932, -143.734788)
  line L106 (48.41323, -139.234115) -> (42.29009, -143.734788)
  spline S86 degree 3 poles (49.189238, -138.049002) (49.189238, -138.528559) (49.019912, -138.782463) (48.41323, -139.234115) knots 0 0 0 0 1 1 1 1
  line L107 (49.189238, -137.964253) -> (49.189238, -138.049002)
  spline S87 degree 3 poles (48.258029, -137.103668) (48.822336, -137.103668) (49.189238, -137.484351) (49.189238, -137.964253) knots 0 0 0 0 1 1 1 1
  line L108 (40.413546, -137.103668) -> (48.258029, -137.103668)
  spline S88 degree 3 poles (44.476864, -125.067193) (47.256367, -125.067193) (49.25969, -127.211765) (49.25969, -130.005049) (49.25969, -132.798677) (47.256367, -134.957373) (44.476864, -134.957373) (41.683409, -134.957373) (39.665788, -132.798677) (39.665788, -130.005049) (39.665788, -127.211765) (41.683409, -125.067193) (44.476864, -125.067193) knots 0 0 0 0 0.25 0.25 0.25 0.5 0.5 0.5 0.75 0.75 0.75 1 1 1 1
  spline S89 degree 3 poles (47.679597, -116.642901) (47.679597, -116.191421) (47.947626, -115.895143) (48.384981, -115.895143) knots 0 0 0 0 1 1 1 1
  line L109 (47.679597, -119.492684) -> (47.679597, -116.642901)
  line L110 (40.413546, -119.492684) -> (47.679597, -119.492684)
  spline S90 degree 3 poles (40.413546, -121.0447) (40.004441, -121.0447) (39.722288, -120.720172) (39.722288, -120.268864) (39.722288, -119.817212) (40.004441, -119.492684) (40.413546, -119.492684) knots 0 0 0 0 0.5 0.5 0.5 1 1 1 1
  line L111 (47.679597, -121.0447) -> (40.413546, -121.0447)
  line L112 (47.679597, -123.866577) -> (47.679597, -121.0447)
  spline S91 degree 3 poles (49.104489, -123.866577) (49.104489, -124.33201) (48.83646, -124.614163) (48.384981, -124.614163) (47.947626, -124.614163) (47.679597, -124.33201) (47.679597, -123.866577) knots 0 0 0 0 0.5 0.5 0.5 1 1 1 1
  line L113 (49.104489, -116.657026) -> (49.104489, -123.866577)
  spline S92 degree 3 poles (48.384981, -115.895143) (48.83646, -115.895143) (49.104489, -116.191421) (49.104489, -116.657026) knots 0 0 0 0 1 1 1 1
  spline S93 degree 3 poles (14.236161, -107.17354) (15.026121, -107.483943) (15.322399, -107.907173) (15.322399, -108.542104) knots 0 0 0 0 1 1 1 1
  line L114 (7.111014, -104.210757) -> (14.236161, -107.17354)
  spline S94 degree 3 poles (6.560832, -104.083633) (6.744456, -104.069681) (6.91361, -104.126008) (7.111014, -104.210757) knots 0 0 0 0 1 1 1 1
  spline S95 degree 3 poles (6.434053, -105.635649) (6.053025, -105.480447) (5.855277, -105.240669) (5.855277, -104.873766) (5.855277, -104.422286) (6.1519, -104.111883) (6.560832, -104.083633) knots 0 0 0 0 0.5 0.5 0.5 1 1 1 1
  line L115 (8.225847, -106.369282) -> (6.434053, -105.635649)
  line L116 (8.225847, -110.785378) -> (8.225847, -106.369282)
  line L117 (6.448178, -111.504886) -> (8.225847, -110.785378)
  spline S96 degree 3 poles (7.054859, -112.986277) (6.871236, -113.056901) (6.716206, -113.099276) (6.603207, -113.099276) (6.166024, -113.099276) (5.855277, -112.746498) (5.855277, -112.280894) (5.855277, -111.942241) (6.06715, -111.660087) (6.448178, -111.504886) knots 0 0 0 0 0.33333333 0.33333333 0.33333333 0.66666667 0.66666667 0.66666667 1 1 1 1
  line L118 (14.236161, -110.023495) -> (7.054859, -112.986277)
  spline S97 degree 3 poles (15.322399, -108.640806) (15.322399, -109.289862) (15.026121, -109.698967) (14.236161, -110.023495) knots 0 0 0 0 1 1 1 1
  line L119 (15.322399, -108.542104) -> (15.322399, -108.640806)
  line L120 (6.673832, -96.520271) -> (14.645093, -96.520271)
  spline S98 degree 3 poles (5.954151, -97.282154) (5.954151, -96.816549) (6.208055, -96.520271) (6.673832, -96.520271) knots 0 0 0 0 1 1 1 1
  line L121 (5.954151, -102.474085) -> (5.954151, -97.282154)
  spline S99 degree 3 poles (7.393167, -102.474085) (7.393167, -102.939689) (7.125139, -103.221843) (6.673832, -103.221843) (6.22218, -103.221843) (5.954151, -102.939689) (5.954151, -102.474085) knots 0 0 0 0 0.5 0.5 0.5 1 1 1 1
  line L122 (7.393167, -98.35444) -> (7.393167, -102.474085)
  spline S100 degree 3 poles (7.717695, -98.072286) (7.463792, -98.072286) (7.393167, -98.156863) (7.393167, -98.35444) knots 0 0 0 0 1 1 1 1
  line L123 (14.645093, -98.072286) -> (7.717695, -98.072286)
  spline S101 degree 3 poles (15.322399, -97.296279) (15.322399, -97.747758) (15.054371, -98.072286) (14.645093, -98.072286) knots 0 0 0 0 1 1 1 1
  spline S102 degree 3 poles (14.645093, -96.520271) (15.054371, -96.520271) (15.322399, -96.844799) (15.322399, -97.296279) knots 0 0 0 0 1 1 1 1
  spline S103 degree 3 poles (13.829639, -74.820476) (11.766027, -74.820476) (10.146832, -75.836434) (10.146832, -79.201776) knots 0 0 0 0 1 1 1 1
  line L124 (27.83068, -74.820476) -> (13.829639, -74.820476)
  line L125 (27.83068, -71.074107) -> (27.83068, -74.820476)
  line L126 (13.797945, -71.074107) -> (27.83068, -71.074107)
  spline S104 degree 3 poles (6.400291, -78.979567) (6.400291, -73.296538) (9.511901, -71.074107) (13.797945, -71.074107) knots 0 0 0 0 1 1 1 1
  line L127 (6.400291, -87.519959) -> (6.400291, -78.979567)
  line L128 (10.146832, -87.519959) -> (6.400291, -87.519959)
  line L129 (10.146832, -79.201776) -> (10.146832, -87.519959)
  line L130 (27.83068, -57.961384) -> (27.83068, -66.850936)
  spline S105 degree 3 poles (20.433198, -50.055923) (24.719242, -50.055923) (27.83068, -52.278355) (27.83068, -57.961384) knots 0 0 0 0 1 1 1 1
  line L131 (6.400291, -50.055923) -> (20.433198, -50.055923)
  line L132 (6.400291, -53.802293) -> (6.400291, -50.055923)
  line L133 (14.877293, -53.802293) -> (6.400291, -53.802293)
  line L134 (14.877293, -66.723984) -> (14.877293, -53.802293)
  line L135 (18.432976, -66.723984) -> (14.877293, -66.723984)
  line L136 (18.432976, -53.802293) -> (18.432976, -66.723984)
  line L137 (20.464893, -53.802293) -> (18.432976, -53.802293)
  spline S106 degree 3 poles (24.084311, -58.215288) (24.084311, -54.818251) (22.465116, -53.802293) (20.464893, -53.802293) knots 0 0 0 0 1 1 1 1
  line L138 (24.084311, -66.850936) -> (24.084311, -58.215288)
  line L139 (27.83068, -66.850936) -> (24.084311, -66.850936)
  line L140 (23.637417, -34.265616) -> (6.397815, -27.471543)
  spline S107 degree 3 poles (23.637417, -36.39279) (24.145569, -36.202276) (24.367778, -35.853116) (24.367778, -35.345136) (24.367778, -34.837157) (24.145569, -34.487996) (23.637417, -34.265616) knots 0 0 0 0 0.5 0.5 0.5 1 1 1 1
  line L141 (6.397815, -42.901264) -> (23.637417, -36.39279)
  line L142 (6.397815, -47.060356) -> (6.397815, -42.901264)
  line L143 (25.447126, -39.821693) -> (6.397815, -47.060356)
  spline S108 degree 3 poles (25.445066, -30.858762) (27.445116, -31.652512) (28.209231, -33.122705) (28.209231, -35.376831) (28.209231, -37.599262) (27.447176, -39.05981) (25.447126, -39.821693) knots 0 0 0 0 0.5 0.5 0.5 1 1 1 1
  line L144 (6.397815, -23.344146) -> (25.445066, -30.858762)
  line L145 (6.397815, -27.471543) -> (6.397815, -23.344146)
  spline S109 degree 3 poles (27.543531, -104.027478) (30.323034, -104.027478) (32.326357, -106.17205) (32.326357, -108.965506) (32.326357, -111.758962) (30.323034, -113.917658) (27.543531, -113.917658) (24.750075, -113.917658) (22.732455, -111.758962) (22.732455, -108.965506) (22.732455, -106.17205) (24.750075, -104.027478) (27.543531, -104.027478) knots 0 0 0 0 0.25 0.25 0.25 0.5 0.5 0.5 0.75 0.75 0.75 1 1 1 1
  line L146 (26.499495, -101.430049) -> (26.499495, -98.072286)
  spline S110 degree 3 poles (27.938511, -101.430049) (27.938511, -101.895653) (27.656358, -102.177807) (27.219003, -102.177807) (26.781648, -102.177807) (26.499495, -101.895653) (26.499495, -101.430049) knots 0 0 0 0 0.5 0.5 0.5 1 1 1 1
  line L147 (27.938511, -98.072286) -> (27.938511, -101.430049)
  line L148 (30.421736, -98.072286) -> (27.938511, -98.072286)
  spline S111 degree 3 poles (30.746264, -98.35444) (30.746264, -98.156863) (30.661515, -98.072286) (30.421736, -98.072286) knots 0 0 0 0 1 1 1 1
  line L149 (30.746264, -102.615161) -> (30.746264, -98.35444)
  spline S112 degree 3 poles (32.171155, -102.601037) (32.171155, -103.066641) (31.903127, -103.348967) (31.451647, -103.348967) (31.014292, -103.348967) (30.746264, -103.066641) (30.746264, -102.615161) knots 0 0 0 0 0.5 0.5 0.5 1 1 1 1
  line L150 (32.171155, -97.225654) -> (32.171155, -102.601037)
  spline S113 degree 3 poles (31.508147, -96.520271) (31.917252, -96.520271) (32.171155, -96.774174) (32.171155, -97.225654) knots 0 0 0 0 1 1 1 1
  line L151 (23.480041, -96.520271) -> (31.508147, -96.520271)
  spline S114 degree 3 poles (23.480041, -98.072286) (23.056983, -98.072286) (22.788955, -97.747758) (22.788955, -97.296279) (22.788955, -96.844799) (23.056983, -96.520271) (23.480041, -96.520271) knots 0 0 0 0 0.5 0.5 0.5 1 1 1 1